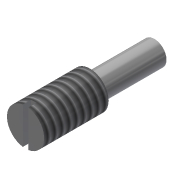
# Autodesk Inventor part: Set_Screw
Saved by Autodesk Inventor 2022 (Build 260148000, 148)
## iProperties
Created: 2006-01-18
Part Number: Set_Screw
Document SubType Name: Modeling
Designer: PMiller
Material: Steel, Mild
Density: 7.85 g/cm^3
Appearance: Steel
Mass: 2.46969 g
Surface Area: 3.28894 cm^2
Volume: 0.31461 cm^3
Author: PMiller
Autodesk Inventor part; units mm, degrees
ref_plane "YZ Plane" through (0, 0, 0) normal (1, 0, 0) x (0, 1, 0)
ref_plane "XZ Plane" through (0, 0, 0) normal (0, 1, 0) x (-1, 0, 0)
ref_plane "XY Plane" through (0, 0, 0) normal (0, 0, 1) x (1, 0, 0)
sketch "Sketch1" plane through (0, 0, 0) normal (0, 0, 1) x (1, 0, 0)
  circle A0 centre (0, 0) radius 2.7432
  dimension "d0" = 5.4864
  constraints: 1 centre point, 1 coincident
  measures "d0" diameter of A0
extrude "Extrusion1" add sketch "Sketch1" against normal blind 9.525
sketch "Sketch2" plane through (0, 0, -9.525) normal (0, 0, -1) x (-1, 0, 0)
  circle A0 centre (0, 0) radius 2.7432 projected
  circle A1 centre (0, 0) radius 1.778
  dimension "d3" = 3.556
  constraints: 1 centre point, 1 coincident
  measures "d3" diameter of A1
extrude "Extrusion2" add sketch "Sketch2" along normal blind 9.525 contours A1
thread "Thread1" size "12-24 UNC" class "2A" standard "ANSI Unified Screw Threads" full length
sketch "Sketch3" plane through (0, 0, 0) normal (0, 0, 1) x (1, 0, 0)
  circle A0 centre (0, 0) radius 2.7432 projected
  line L0 (-0.3969, 2.7143) -> (-0.3969, -2.7143)
  line L1 (0.3969, -2.7143) -> (0.3969, 2.7143)
  dimension "d8" = 0.7937
  dimension "d9" = 0.3969
  constraints: 4 end point, 4 point on circle, 1 parallel, 1 vertical
  measures "d8" distance between parallel lines of L1 L0
  measures "d9" distance from line of A0.centre L0
extrude "Extrusion3" cut sketch "Sketch3" against normal blind 1.1906 contours L1 A0 L0
equation "\"d9\" = 0.5 * d8"
body "Solid1"
